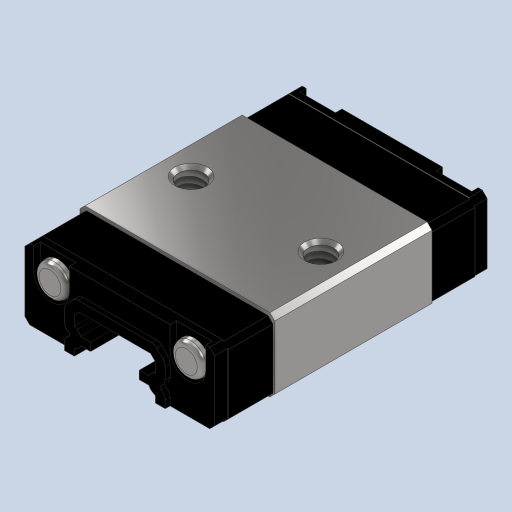
# Autodesk Inventor part: SSEB6_b
Saved by Autodesk Inventor 2023 (Build 270158000, 158)
## iProperties
Category: PARTsolutions
Company: MISUMI
Created: 2024-12-17
Part Number: SSEB6_b
Material: ステンレス鋼
Catalog Web Link: www.cadenas.de
Description: SSEB, SSEB-MX, SSEBV, SSEBV-MX, SSE2B, SSE2B-MX, SSE2BV, SSE2BV-MX, SSEBL, SSEBL-MX, SSEBLV, SSEBLV-MX, SSE2BL, SSE2BL-MX, SSE2BLV, SSE2BLV-MX, SEB, SEBV, SE2B, SE2BV, SEBL, SEBLV, SE2BL, SE2BLV_block-Miniature Linear Guides - Short Block, Standard Preload - High/Precision Grade
Vendor: MISUMI
Document SubType Name: Modeling
Designer: psAdmin
Manufacturer: MISUMI
Mass: 5.50515 g
Surface Area: 8.12596 cm^2
Volume: 0.688144 cm^3
Density: 8 g/cm^3
Appearance: 半つや出し
PSOL_IDENT_0: {$CADENAS_DATA/23d-libs/misumi/metric/06_linear_guides/seb_series/seb_block.prj},358 {VTYP=3D},{NB=S
PSOL_IDENT_1: SEB6_b},{LINA=SSEB6},{NN=SSEB, SSEB-MX, SSEBV, SSEBV-MX, SSE2B, SSE2B-MX, SSE2BV, SSE2BV-MX, SSEBL,
PSOL_IDENT_2: SSEBL-MX, SSEBLV, SSEBLV-MX, SSE2BL, SSE2BL-MX, SSE2BLV, SSE2BLV-MX, SEB, SEBV, SE2B, SE2BV, SEBL, S
PSOL_IDENT_3: EBLV, SE2BL, SE2BLV_block},{DATE=01.06.2021 05:33:03},{GEOMDATE=29.09.2020 01:45:00},{VERSION=},{LIN
PSOL_IDENT_4: EID=60},{WBVAR=TS,MAT,ST,MX},{WBNUMERIC=}  {NB=SSEB6_b},{LINA=SSEB6},{KT=DUMMY},{PN=SSEB6},{TS=},{TY
PSOL_IDENT_5: PE=SSEB},{H=6},{MAT=S},{ST=S},{ST1='S', 'w/o Surface Treatment'},{HARD=56HRC~},{STPN=S},{MX=},{MXALG=
PSOL_IDENT_6: '','w/o MX(Lubrication unit)' },{W=12},{L1=17.4},{B=8},{C=0},{SLL=M2x1.5},{S=2},{LL=1.5},{L2=9.7},{
PSOL_IDENT_7: K=4.5},{CBB=0.3},{W1=5},{W2=3.5},{H1=4.0},{CAA=0.3},{F=15},{G=5.0},{CA1=0.3},{CA2=0.3},{VA1=1.5},{HA
PSOL_IDENT_8: 1=1.0},{WA1=1.2167},{WA2=0.5},{RA1=1.00},{HA2=5.1372},{POIA1=-0.1473},{BHA1=8.4},{BHA2=11.7},{BHA3=1
PSOL_IDENT_9: 1.8},{BHA5=0.0000},{BHA6=0.0},{BHA7=0.0},{BHA8=0.0},{BVA1=1.52},{BVA3=0.15},{BVA4=0.15},{BVA5=4.35},
PSOL_IDENT_10: {BVA6=4.35},{BCA1=0.3},{BCA2H=0.0},{BCA2V=0.00},{BRA1=1.10},{BRA2=1.00},{BDA1=0.00},{BHB1=6.2064},{B
PSOL_IDENT_11: HB2=5.1826},{BVB1=3.1032},{BVB2=1.0652},{BRB1=0.0},{BRB2=0.4732},{BRB3=0.3},{BHC1=2.75},{BHC2=0.8},{
PSOL_IDENT_12: BHC3=0.5},{BHC4=0.4},{BHC5=0.3},{MD=2.3}
NB: SSEB6_b
NN: SSEB, SSEB-MX, SSEBV, SSEBV-MX, SSE2B, SSE2B-MX, SSE2BV, SSE2BV-MX, SSEBL, SSEBL-MX, SSEBLV, SSEBLV-MX, SSE2BL, SSE2BL-MX, SSE2BLV, SSE2BLV-MX, SEB, SEBV, SE2B, SE2BV, SEBL, SEBLV, SE2BL, SE2BLV_block
NT: Miniature Linear Guides - Short Block, Standard Preload - High/Precision Grade
NBSYN: $PN._b
LINA: SSEB6
CATALOG: Misumi
PN: SSEB6
TS: Advanced
H: 6
MAT: Stainless Steel
ST: w/o Surface Treatment
MX: w/o MX(Lubrication unit)
W: 12
L1: 17.4
B: 8
C: 0
SLL: M2x1.5
S: 2
LL: 1.5
L2: 9.7
K: 4.5
CBB: 0.3
W1: 5
W2: 3.5
H1: 4
CAA: 0.3
F: 15
G: 5
CA1: 0.3
CA2: 0.3
VA1: 1.5
HA1: 1
WA1: 1.2167
WA2: 0.5
RA1: 1
HA2: 5.1372
POIA1: -0.1473
BHA1: 8.4
BHA2: 11.7
BHA3: 11.8
BHA5: 0
BHA6: 0
BHA7: 0
BHA8: 0
BVA1: 1.52
BVA3: 0.15
BVA4: 0.15
BVA5: 4.35
BVA6: 4.35
BCA1: 0.3
BCA2H: 0
BCA2V: 0
BRA1: 1.1
BRA2: 1
BDA1: 0
BHB1: 6.2064
BHB2: 5.1826
BVB1: 3.1032
BVB2: 1.0652
BRB1: 0
BRB2: 0.4732
BRB3: 0.3
BHC1: 2.75
BHC2: 0.8
BHC3: 0.5
BHC4: 0.4
BHC5: 0.3
MD: 2.3
SUPPLIER: MISUMI
ARTICLENO: SSEB6_b
BOMINFO: SSEB6
CREATOR: CADENAS GmbH
Title: SSEB6
Author: Cadenas PARTsolutions
Comments: Miniature Linear Guides - Short Block, Standard Preload - High/Precision Grade
Autodesk Inventor part; units mm, degrees
sketch "Sketch_29" plane through (0, 0, 0) normal (0, 0, 1) x (1, 0, 0)
  line L0 (-6, 1.8) -> (-5.7, 1.5)
  line L1 (-5.7, 1.5) -> (5.7, 1.5)
  line L2 (5.7, 1.5) -> (6, 1.8)
  line L3 (6, 1.8) -> (6, 5.7)
  line L4 (6, 5.7) -> (5.7, 6)
  line L5 (5.7, 6) -> (-5.7, 6)
  line L6 (-5.7, 6) -> (-6, 5.7)
  line L7 (-6, 5.7) -> (-6, 1.8)
  constraints: 16 end point
extrude "Extrusion1" add sketch "Sketch_29" along normal mid plane 9.7
sketch "Sketch_3" plane through (0, 0, 4.85) normal (0, 0, 1) x (1, 0, 0)
  line L0 (-5.9, 5.55) -> (-5.9, 1.8)
  line L1 (-5.9, 1.8) -> (-5.6, 1.5)
  line L2 (-5.6, 1.5) -> (5.6, 1.5)
  line L3 (5.6, 1.5) -> (5.9, 1.8)
  line L4 (5.9, 1.8) -> (5.9, 5.55)
  line L5 (5.9, 5.55) -> (5.6, 5.85)
  line L6 (5.6, 5.85) -> (-5.6, 5.85)
  line L7 (-5.6, 5.85) -> (-5.9, 5.55)
  constraints: 16 end point
extrude "Extrusion2" add sketch "Sketch_3" along normal blind 3.85
sketch "Sketch_42" plane through (0, 0, 4.85) normal (0, 0, 1) x (1, 0, 0)
  line L0 (-12, 7.2) -> (-12, 0)
  line L1 (-12, 0) -> (12, 0)
  line L2 (12, 0) -> (12, 7.2)
  line L3 (12, 7.2) -> (-12, 7.2)
  line L4 (-5.9, 5.5) -> (-5.9, 1.8)
  line L5 (-5.9, 1.8) -> (-5.6, 1.5)
  line L6 (-5.6, 1.5) -> (5.6, 1.5)
  line L7 (5.6, 1.5) -> (5.9, 1.8)
  line L8 (5.9, 1.8) -> (5.9, 5.5)
  line L9 (5.9, 5.5) -> (5.6, 5.8)
  line L10 (5.6, 5.8) -> (-5.6, 5.8)
  line L11 (-5.6, 5.8) -> (-5.9, 5.5)
  constraints: 24 end point
extrude "Extrusion3" cut sketch "Sketch_42" along normal blind 2.75
sketch "Sketch_4" plane through (0, 0, -4.85) normal (0, 0, 1) x (1, 0, 0)
  line L0 (-5.9, 5.55) -> (-5.9, 1.8)
  line L1 (-5.9, 1.8) -> (-5.6, 1.5)
  line L2 (-5.6, 1.5) -> (5.6, 1.5)
  line L3 (5.6, 1.5) -> (5.9, 1.8)
  line L4 (5.9, 1.8) -> (5.9, 5.55)
  line L5 (5.9, 5.55) -> (5.6, 5.85)
  line L6 (5.6, 5.85) -> (-5.6, 5.85)
  line L7 (-5.6, 5.85) -> (-5.9, 5.55)
  constraints: 16 end point
extrude "Extrusion4" add sketch "Sketch_4" against normal blind 3.85
sketch "Sketch_43" plane through (0, 0, -4.85) normal (0, 0, 1) x (1, 0, 0)
  line L0 (-12, 7.2) -> (-12, 0)
  line L1 (-12, 0) -> (12, 0)
  line L2 (12, 0) -> (12, 7.2)
  line L3 (12, 7.2) -> (-12, 7.2)
  line L4 (-5.9, 5.5) -> (-5.9, 1.8)
  line L5 (-5.9, 1.8) -> (-5.6, 1.5)
  line L6 (-5.6, 1.5) -> (5.6, 1.5)
  line L7 (5.6, 1.5) -> (5.9, 1.8)
  line L8 (5.9, 1.8) -> (5.9, 5.5)
  line L9 (5.9, 5.5) -> (5.6, 5.8)
  line L10 (5.6, 5.8) -> (-5.6, 5.8)
  line L11 (-5.6, 5.8) -> (-5.9, 5.5)
  constraints: 24 end point
extrude "Extrusion5" cut sketch "Sketch_43" against normal blind 2.75
sketch "Sketch_30" plane through (0, 0, 8.7) normal (0, 0, 1) x (1, 0, 0)
  line L0 (-12, 9) -> (-12, 0)
  line L1 (-12, 0) -> (12, 0)
  line L2 (12, 0) -> (12, 9)
  line L3 (12, 9) -> (-12, 9)
  line L4 (-5.85, 1.8) -> (-5.55, 1.5)
  line L5 (-5.55, 1.5) -> (5.55, 1.5)
  line L6 (5.55, 1.5) -> (5.85, 1.8)
  line L7 (5.85, 1.8) -> (5.85, 5.55)
  line L8 (5.85, 5.55) -> (5.55, 5.85)
  line L9 (5.55, 5.85) -> (5.3, 5.85)
  line L10 (5.3, 5.85) -> (5.3, 4.48)
  arc A0 (3.1, 4.48) -> (5.3, 4.48) centre (4.2, 4.48) ccw
  line L11 (3.1, 4.48) -> (3.1, 5.85)
  line L12 (3.1, 5.85) -> (-3.1, 5.85)
  line L13 (-3.1, 5.85) -> (-3.1, 4.48)
  arc A1 (-5.3, 4.48) -> (-3.1, 4.48) centre (-4.2, 4.48) ccw
  line L14 (-5.3, 4.48) -> (-5.3, 5.85)
  line L15 (-5.3, 5.85) -> (-5.55, 5.85)
  line L16 (-5.55, 5.85) -> (-5.85, 5.55)
  line L17 (-5.85, 5.55) -> (-5.85, 1.8)
  constraints: 36 end point, 4 point on circle, 2 centre point
extrude "Extrusion6" cut sketch "Sketch_30" against normal blind 1.1
sketch "_____2" plane through (0, 0, 8.7) normal (0, 0, 1) x (1, 0, 0)
  line L0 (-12, 7.2) -> (-12, 0)
  line L1 (-12, 0) -> (-3.1032, 0)
  line L2 (-3.1032, 0) -> (-3.1032, 1.9674)
  arc A0 (-2.8479, 2.3874) -> (-3.1032, 1.9674) centre (-2.63, 1.9674) ccw
  arc A1 (-2.8479, 2.3874) -> (-2.8479, 2.6126) centre (-2.9063, 2.5) ccw
  arc A2 (-3.1032, 3.0326) -> (-2.8479, 2.6126) centre (-2.63, 3.0326) ccw
  line L3 (-3.1032, 3.0326) -> (-3.1032, 3.7539)
  arc A3 (-2.9646, 4.0885) -> (-3.1032, 3.7539) centre (-2.63, 3.7539) ccw
  line L4 (-2.9646, 4.0885) -> (-2.5885, 4.4646)
  arc A4 (-2.2539, 4.6032) -> (-2.5885, 4.4646) centre (-2.2539, 4.13) ccw
  line L5 (-2.2539, 4.6032) -> (2.2539, 4.6032)
  arc A5 (2.5885, 4.4646) -> (2.2539, 4.6032) centre (2.2539, 4.13) ccw
  line L6 (2.5885, 4.4646) -> (2.9646, 4.0885)
  arc A6 (3.1032, 3.7539) -> (2.9646, 4.0885) centre (2.63, 3.7539) ccw
  line L7 (3.1032, 3.7539) -> (3.1032, 3.0326)
  arc A7 (2.8479, 2.6126) -> (3.1032, 3.0326) centre (2.63, 3.0326) ccw
  arc A8 (2.8479, 2.6126) -> (2.8479, 2.3874) centre (2.9063, 2.5) ccw
  arc A9 (3.1032, 1.9674) -> (2.8479, 2.3874) centre (2.63, 1.9674) ccw
  line L8 (3.1032, 1.9674) -> (3.1032, 0)
  line L9 (3.1032, 0) -> (12, 0)
  line L10 (12, 0) -> (12, 7.2)
  line L11 (12, 7.2) -> (-12, 7.2)
  constraints: 24 end point, 20 point on circle, 10 centre point
extrude "Extrusion7" cut sketch "_____2" against normal blind 0.3
sketch "Sketch_31" plane through (0, 0, -8.7) normal (0, 0, 1) x (1, 0, 0)
  line L0 (-12, 9) -> (-12, 0)
  line L1 (-12, 0) -> (12, 0)
  line L2 (12, 0) -> (12, 9)
  line L3 (12, 9) -> (-12, 9)
  line L4 (-5.85, 1.8) -> (-5.55, 1.5)
  line L5 (-5.55, 1.5) -> (5.55, 1.5)
  line L6 (5.55, 1.5) -> (5.85, 1.8)
  line L7 (5.85, 1.8) -> (5.85, 5.55)
  line L8 (5.85, 5.55) -> (5.55, 5.85)
  line L9 (5.55, 5.85) -> (5.3, 5.85)
  line L10 (5.3, 5.85) -> (5.3, 4.48)
  arc A0 (3.1, 4.48) -> (5.3, 4.48) centre (4.2, 4.48) ccw
  line L11 (3.1, 4.48) -> (3.1, 5.85)
  line L12 (3.1, 5.85) -> (-3.1, 5.85)
  line L13 (-3.1, 5.85) -> (-3.1, 4.48)
  arc A1 (-5.3, 4.48) -> (-3.1, 4.48) centre (-4.2, 4.48) ccw
  line L14 (-5.3, 4.48) -> (-5.3, 5.85)
  line L15 (-5.3, 5.85) -> (-5.55, 5.85)
  line L16 (-5.55, 5.85) -> (-5.85, 5.55)
  line L17 (-5.85, 5.55) -> (-5.85, 1.8)
  constraints: 36 end point, 4 point on circle, 2 centre point
extrude "Extrusion8" cut sketch "Sketch_31" along normal blind 1.1
sketch "_____1" plane through (0, 0, -8.7) normal (0, 0, 1) x (1, 0, 0)
  line L0 (-12, 7.2) -> (-12, 0)
  line L1 (-12, 0) -> (-3.1032, 0)
  line L2 (-3.1032, 0) -> (-3.1032, 1.9674)
  arc A0 (-2.8479, 2.3874) -> (-3.1032, 1.9674) centre (-2.63, 1.9674) ccw
  arc A1 (-2.8479, 2.3874) -> (-2.8479, 2.6126) centre (-2.9063, 2.5) ccw
  arc A2 (-3.1032, 3.0326) -> (-2.8479, 2.6126) centre (-2.63, 3.0326) ccw
  line L3 (-3.1032, 3.0326) -> (-3.1032, 3.7539)
  arc A3 (-2.9646, 4.0885) -> (-3.1032, 3.7539) centre (-2.63, 3.7539) ccw
  line L4 (-2.9646, 4.0885) -> (-2.5885, 4.4646)
  arc A4 (-2.2539, 4.6032) -> (-2.5885, 4.4646) centre (-2.2539, 4.13) ccw
  line L5 (-2.2539, 4.6032) -> (2.2539, 4.6032)
  arc A5 (2.5885, 4.4646) -> (2.2539, 4.6032) centre (2.2539, 4.13) ccw
  line L6 (2.5885, 4.4646) -> (2.9646, 4.0885)
  arc A6 (3.1032, 3.7539) -> (2.9646, 4.0885) centre (2.63, 3.7539) ccw
  line L7 (3.1032, 3.7539) -> (3.1032, 3.0326)
  arc A7 (2.8479, 2.6126) -> (3.1032, 3.0326) centre (2.63, 3.0326) ccw
  arc A8 (2.8479, 2.6126) -> (2.8479, 2.3874) centre (2.9063, 2.5) ccw
  arc A9 (3.1032, 1.9674) -> (2.8479, 2.3874) centre (2.63, 1.9674) ccw
  line L8 (3.1032, 1.9674) -> (3.1032, 0)
  line L9 (3.1032, 0) -> (12, 0)
  line L10 (12, 0) -> (12, 7.2)
  line L11 (12, 7.2) -> (-12, 7.2)
  constraints: 24 end point, 20 point on circle, 10 centre point
extrude "Extrusion9" cut sketch "_____1" along normal blind 0.3
sketch "Sketch_32" plane through (0, 0, 7.6) normal (0, 0, 1) x (1, 0, 0)
  arc A0 (-5.3, 4.48) -> (-3.1, 4.48) centre (-4.2, 4.48) ccw
  line L0 (-3.1, 4.48) -> (-3.1, 5.85)
  line L1 (-3.1, 5.85) -> (-5.3, 5.85)
  line L2 (-5.3, 5.85) -> (-5.3, 4.48)
  constraints: 6 end point, 2 point on circle, 1 centre point
extrude "Extrusion10" add sketch "Sketch_32" along normal blind 0.4
sketch "Sketch_33" plane through (0, 0, 7.6) normal (0, 0, 1) x (1, 0, 0)
  arc A0 (3.1, 4.48) -> (5.3, 4.48) centre (4.2, 4.48) ccw
  line L0 (5.3, 4.48) -> (5.3, 5.85)
  line L1 (5.3, 5.85) -> (3.1, 5.85)
  line L2 (3.1, 5.85) -> (3.1, 4.48)
  constraints: 6 end point, 2 point on circle, 1 centre point
extrude "Extrusion11" add sketch "Sketch_33" along normal blind 0.4
sketch "Sketch_34" plane through (0, 0, -7.6) normal (0, 0, 1) x (1, 0, 0)
  arc A0 (-5.3, 4.48) -> (-3.1, 4.48) centre (-4.2, 4.48) ccw
  line L0 (-3.1, 4.48) -> (-3.1, 5.85)
  line L1 (-3.1, 5.85) -> (-5.3, 5.85)
  line L2 (-5.3, 5.85) -> (-5.3, 4.48)
  constraints: 6 end point, 2 point on circle, 1 centre point
extrude "Extrusion12" add sketch "Sketch_34" against normal blind 0.4
sketch "Sketch_35" plane through (0, 0, -7.6) normal (0, 0, 1) x (1, 0, 0)
  arc A0 (3.1, 4.48) -> (5.3, 4.48) centre (4.2, 4.48) ccw
  line L0 (5.3, 4.48) -> (5.3, 5.85)
  line L1 (5.3, 5.85) -> (3.1, 5.85)
  line L2 (3.1, 5.85) -> (3.1, 4.48)
  constraints: 6 end point, 2 point on circle, 1 centre point
extrude "Extrusion13" add sketch "Sketch_35" against normal blind 0.4
sketch "Sketch_36" plane through (-4.2, 0, 0) normal (1, 0, 0) x (0, 0, -1)
  line L0 (-8, 4.48) -> (-8.5, 4.48)
  line L1 (-8.5, 4.48) -> (-8.5, 5.1602)
  arc A0 (-8.2277, 5.4589) -> (-8.5, 5.1602) centre (-8.2, 5.1602) ccw
  line L2 (-8.2277, 5.4589) -> (-8, 5.48)
  line L3 (-8, 5.48) -> (-8, 4.48)
  line L4 (-8, 4.48) -> (-8.5, 4.48)
  constraints: 10 end point, 2 point on circle, 1 centre point
revolve "Revolution1" add sketch "Sketch_36" angle 360 about axis through (-4.2, 4.48, 8) along (0, 0, -1)
sketch "Sketch_37" plane through (-4.2, 0, 0) normal (1, 0, 0) x (0, 0, -1)
  line L0 (8.5, 4.48) -> (8, 4.48)
  line L1 (8, 4.48) -> (8, 5.48)
  line L2 (8, 5.48) -> (8.2277, 5.4589)
  arc A0 (8.5, 5.1602) -> (8.2277, 5.4589) centre (8.2, 5.1602) ccw
  line L3 (8.5, 5.1602) -> (8.5, 4.48)
  line L4 (8.5, 4.48) -> (8, 4.48)
  constraints: 10 end point, 2 point on circle, 1 centre point
revolve "Revolution2" add sketch "Sketch_37" angle 360 about axis through (-4.2, 4.48, -8.5) along (0, 0, -1)
sketch "Sketch_38" plane through (4.2, 0, 0) normal (1, 0, 0) x (0, 0, -1)
  line L0 (-8, 4.48) -> (-8.5, 4.48)
  line L1 (-8.5, 4.48) -> (-8.5, 5.1602)
  arc A0 (-8.2277, 5.4589) -> (-8.5, 5.1602) centre (-8.2, 5.1602) ccw
  line L2 (-8.2277, 5.4589) -> (-8, 5.48)
  line L3 (-8, 5.48) -> (-8, 4.48)
  line L4 (-8, 4.48) -> (-8.5, 4.48)
  constraints: 10 end point, 2 point on circle, 1 centre point
revolve "Revolution3" add sketch "Sketch_38" angle 360 about axis through (4.2, 4.48, 8) along (0, 0, -1)
sketch "Sketch_39" plane through (4.2, 0, 0) normal (1, 0, 0) x (0, 0, -1)
  line L0 (8.5, 4.48) -> (8, 4.48)
  line L1 (8, 4.48) -> (8, 5.48)
  line L2 (8, 5.48) -> (8.2277, 5.4589)
  arc A0 (8.5, 5.1602) -> (8.2277, 5.4589) centre (8.2, 5.1602) ccw
  line L3 (8.5, 5.1602) -> (8.5, 4.48)
  line L4 (8.5, 4.48) -> (8, 4.48)
  constraints: 10 end point, 2 point on circle, 1 centre point
revolve "Revolution4" add sketch "Sketch_39" angle 360 about axis through (4.2, 4.48, -8.5) along (0, 0, -1)
sketch "Sketch_17" plane through (0, 0, 0) normal (0, 0, 1) x (1, 0, 0)
  line L0 (-2.5, 3.7) -> (-2.5, 3.1084)
  line L1 (-2.5, 3.1084) -> (-2.3242, 3.0098)
  arc A0 (-2.1007, 2.75) -> (-2.3242, 3.0098) centre (-2.5686, 2.5736) ccw
  line L2 (-2.1007, 2.75) -> (-1.5, 2.75)
  line L3 (-1.5, 2.75) -> (-1.5, 2.25)
  line L4 (-1.5, 2.25) -> (-2.1007, 2.25)
  arc A1 (-2.3242, 1.9902) -> (-2.1007, 2.25) centre (-2.5686, 2.4264) ccw
  line L5 (-2.3242, 1.9902) -> (-2.5, 1.8917)
  line L6 (-2.5, 1.8917) -> (-2.5, 0.3)
  line L7 (-2.5, 0.3) -> (-2.2, 0)
  line L8 (-2.2, 0) -> (2.2, 0)
  line L9 (2.2, 0) -> (2.5, 0.3)
  line L10 (2.5, 0.3) -> (2.5, 1.8917)
  line L11 (2.5, 1.8917) -> (2.3242, 1.9902)
  arc A2 (2.1007, 2.25) -> (2.3242, 1.9902) centre (2.5686, 2.4263) ccw
  line L12 (2.1007, 2.25) -> (1.5, 2.25)
  line L13 (1.5, 2.25) -> (1.5, 2.75)
  line L14 (1.5, 2.75) -> (2.1007, 2.75)
  arc A3 (2.3242, 3.0098) -> (2.1007, 2.75) centre (2.5686, 2.5737) ccw
  line L15 (2.3242, 3.0098) -> (2.5, 3.1084)
  line L16 (2.5, 3.1084) -> (2.5, 3.7)
  line L17 (2.5, 3.7) -> (2.2, 4)
  line L18 (2.2, 4) -> (-2.2, 4)
  line L19 (-2.2, 4) -> (-2.5, 3.7)
  constraints: 40 end point, 8 point on circle, 4 centre point
extrude "Extrusion14" cut sketch "Sketch_17" along normal mid plane 9.7
sketch "Sketch_11" plane through (0, 0, 4.85) normal (0, 0, 1) x (1, 0, 0)
  line L0 (-2.5, 3.7) -> (-2.5, 3.1084)
  line L1 (-2.5, 3.1084) -> (-2.3242, 3.0098)
  arc A0 (-2.1007, 2.75) -> (-2.3242, 3.0098) centre (-2.5686, 2.5736) ccw
  line L2 (-2.1007, 2.75) -> (-1.5, 2.75)
  line L3 (-1.5, 2.75) -> (-1.5, 2.25)
  line L4 (-1.5, 2.25) -> (-2.1007, 2.25)
  arc A1 (-2.3242, 1.9902) -> (-2.1007, 2.25) centre (-2.5686, 2.4264) ccw
  line L5 (-2.3242, 1.9902) -> (-2.5, 1.8917)
  line L6 (-2.5, 1.8917) -> (-2.5, 0.3)
  line L7 (-2.5, 0.3) -> (-2.2, 0)
  line L8 (-2.2, 0) -> (2.2, 0)
  line L9 (2.2, 0) -> (2.5, 0.3)
  line L10 (2.5, 0.3) -> (2.5, 1.8917)
  line L11 (2.5, 1.8917) -> (2.3242, 1.9902)
  arc A2 (2.1007, 2.25) -> (2.3242, 1.9902) centre (2.5686, 2.4263) ccw
  line L12 (2.1007, 2.25) -> (1.5, 2.25)
  line L13 (1.5, 2.25) -> (1.5, 2.75)
  line L14 (1.5, 2.75) -> (2.1007, 2.75)
  arc A3 (2.3242, 3.0098) -> (2.1007, 2.75) centre (2.5686, 2.5737) ccw
  line L15 (2.3242, 3.0098) -> (2.5, 3.1084)
  line L16 (2.5, 3.1084) -> (2.5, 3.7)
  line L17 (2.5, 3.7) -> (2.2, 4)
  line L18 (2.2, 4) -> (-2.2, 4)
  line L19 (-2.2, 4) -> (-2.5, 3.7)
  constraints: 40 end point, 8 point on circle, 4 centre point
extrude "Extrusion15" cut sketch "Sketch_11" along normal blind 4.85
sketch "Sketch_22" plane through (0, 0, 4.85) normal (0, 0, 1) x (1, 0, 0)
  line L0 (-12, 9) -> (-12, 0)
  line L1 (-12, 0) -> (12, 0)
  line L2 (12, 0) -> (12, 9)
  line L3 (12, 9) -> (-12, 9)
  line L4 (-5.9, 5.6) -> (-5.9, 1.8)
  line L5 (-5.9, 1.8) -> (-5.65, 1.55)
  line L6 (-5.65, 1.55) -> (-2.55, 1.55)
  line L7 (-2.55, 1.55) -> (-2.55, 1.9417)
  line L8 (-2.55, 1.9417) -> (-2.3847, 2.0156)
  arc A0 (-2.3847, 2.0156) -> (-2.1367, 2.3) centre (-2.5686, 2.4263) ccw
  line L9 (-2.1367, 2.3) -> (-1.55, 2.3)
  line L10 (-1.55, 2.3) -> (-1.55, 2.7)
  line L11 (-1.55, 2.7) -> (-2.1367, 2.7)
  arc A1 (-2.1367, 2.7) -> (-2.3847, 2.9844) centre (-2.5686, 2.5737) ccw
  line L12 (-2.3847, 2.9844) -> (-2.55, 3.0584)
  line L13 (-2.55, 3.0584) -> (-2.55, 3.75)
  line L14 (-2.55, 3.75) -> (-2.25, 4.05)
  line L15 (-2.25, 4.05) -> (2.25, 4.05)
  line L16 (2.25, 4.05) -> (2.55, 3.75)
  line L17 (2.55, 3.75) -> (2.55, 3.0584)
  line L18 (2.55, 3.0584) -> (2.3847, 2.9844)
  arc A2 (2.3847, 2.9844) -> (2.1367, 2.7) centre (2.5686, 2.5737) ccw
  line L19 (2.1367, 2.7) -> (1.55, 2.7)
  line L20 (1.55, 2.7) -> (1.55, 2.3)
  line L21 (1.55, 2.3) -> (2.1367, 2.3)
  arc A3 (2.1367, 2.3) -> (2.3847, 2.0156) centre (2.5686, 2.4263) ccw
  line L22 (2.3847, 2.0156) -> (2.55, 1.9417)
  line L23 (2.55, 1.9417) -> (2.55, 1.55)
  line L24 (2.55, 1.55) -> (5.65, 1.55)
  line L25 (5.65, 1.55) -> (5.9, 1.8)
  line L26 (5.9, 1.8) -> (5.9, 5.6)
  line L27 (5.9, 5.6) -> (5.65, 5.85)
  line L28 (5.65, 5.85) -> (-5.65, 5.85)
  line L29 (-5.65, 5.85) -> (-5.9, 5.6)
  constraints: 60 end point, 8 point on circle, 4 centre point
extrude "Extrusion16" cut sketch "Sketch_22" along normal blind 0.05
sketch "Sketch_10" plane through (0, 0, -4.85) normal (0, 0, 1) x (1, 0, 0)
  line L0 (-2.5, 3.7) -> (-2.5, 3.1084)
  line L1 (-2.5, 3.1084) -> (-2.3242, 3.0098)
  arc A0 (-2.1007, 2.75) -> (-2.3242, 3.0098) centre (-2.5686, 2.5736) ccw
  line L2 (-2.1007, 2.75) -> (-1.5, 2.75)
  line L3 (-1.5, 2.75) -> (-1.5, 2.25)
  line L4 (-1.5, 2.25) -> (-2.1007, 2.25)
  arc A1 (-2.3242, 1.9902) -> (-2.1007, 2.25) centre (-2.5686, 2.4264) ccw
  line L5 (-2.3242, 1.9902) -> (-2.5, 1.8917)
  line L6 (-2.5, 1.8917) -> (-2.5, 0.3)
  line L7 (-2.5, 0.3) -> (-2.2, 0)
  line L8 (-2.2, 0) -> (2.2, 0)
  line L9 (2.2, 0) -> (2.5, 0.3)
  line L10 (2.5, 0.3) -> (2.5, 1.8917)
  line L11 (2.5, 1.8917) -> (2.3242, 1.9902)
  arc A2 (2.1007, 2.25) -> (2.3242, 1.9902) centre (2.5686, 2.4263) ccw
  line L12 (2.1007, 2.25) -> (1.5, 2.25)
  line L13 (1.5, 2.25) -> (1.5, 2.75)
  line L14 (1.5, 2.75) -> (2.1007, 2.75)
  arc A3 (2.3242, 3.0098) -> (2.1007, 2.75) centre (2.5686, 2.5737) ccw
  line L15 (2.3242, 3.0098) -> (2.5, 3.1084)
  line L16 (2.5, 3.1084) -> (2.5, 3.7)
  line L17 (2.5, 3.7) -> (2.2, 4)
  line L18 (2.2, 4) -> (-2.2, 4)
  line L19 (-2.2, 4) -> (-2.5, 3.7)
  constraints: 40 end point, 8 point on circle, 4 centre point
extrude "Extrusion17" cut sketch "Sketch_10" against normal blind 4.85
sketch "Sketch_23" plane through (0, 0, -4.85) normal (0, 0, 1) x (1, 0, 0)
  line L0 (-12, 9) -> (-12, 0)
  line L1 (-12, 0) -> (12, 0)
  line L2 (12, 0) -> (12, 9)
  line L3 (12, 9) -> (-12, 9)
  line L4 (-5.9, 5.6) -> (-5.9, 1.8)
  line L5 (-5.9, 1.8) -> (-5.65, 1.55)
  line L6 (-5.65, 1.55) -> (-2.55, 1.55)
  line L7 (-2.55, 1.55) -> (-2.55, 1.9417)
  line L8 (-2.55, 1.9417) -> (-2.3847, 2.0156)
  arc A0 (-2.3847, 2.0156) -> (-2.1367, 2.3) centre (-2.5686, 2.4263) ccw
  line L9 (-2.1367, 2.3) -> (-1.55, 2.3)
  line L10 (-1.55, 2.3) -> (-1.55, 2.7)
  line L11 (-1.55, 2.7) -> (-2.1367, 2.7)
  arc A1 (-2.1367, 2.7) -> (-2.3847, 2.9844) centre (-2.5686, 2.5737) ccw
  line L12 (-2.3847, 2.9844) -> (-2.55, 3.0584)
  line L13 (-2.55, 3.0584) -> (-2.55, 3.75)
  line L14 (-2.55, 3.75) -> (-2.25, 4.05)
  line L15 (-2.25, 4.05) -> (2.25, 4.05)
  line L16 (2.25, 4.05) -> (2.55, 3.75)
  line L17 (2.55, 3.75) -> (2.55, 3.0584)
  line L18 (2.55, 3.0584) -> (2.3847, 2.9844)
  arc A2 (2.3847, 2.9844) -> (2.1367, 2.7) centre (2.5686, 2.5737) ccw
  line L19 (2.1367, 2.7) -> (1.55, 2.7)
  line L20 (1.55, 2.7) -> (1.55, 2.3)
  line L21 (1.55, 2.3) -> (2.1367, 2.3)
  arc A3 (2.1367, 2.3) -> (2.3847, 2.0156) centre (2.5686, 2.4263) ccw
  line L22 (2.3847, 2.0156) -> (2.55, 1.9417)
  line L23 (2.55, 1.9417) -> (2.55, 1.55)
  line L24 (2.55, 1.55) -> (5.65, 1.55)
  line L25 (5.65, 1.55) -> (5.9, 1.8)
  line L26 (5.9, 1.8) -> (5.9, 5.6)
  line L27 (5.9, 5.6) -> (5.65, 5.85)
  line L28 (5.65, 5.85) -> (-5.65, 5.85)
  line L29 (-5.65, 5.85) -> (-5.9, 5.6)
  constraints: 60 end point, 8 point on circle, 4 centre point
extrude "Extrusion18" cut sketch "Sketch_23" against normal blind 0.05
sketch "Sketch23" plane through (-5.7, 6, 4.85) normal (0, 1, 0) x (1, 0, 0)
  point P0 (1.7, 4.85)
hole "Hole1" at (-4, 6, 0) direction (0, -1, 0) diameter 1.567 depth 2.3 tip angle 120 countersink diameter 2 countersink angle 90 thread size "M2x0.4" class "6H" standard "ISO Metric profile"
pattern_linear "Rectangular Pattern1" count 2 spacing 8 along (1, 0, 0) of "Hole1"
ref_plane "to_rail_XY" through (0, 4, 0) normal (0, 0, 1) x (1, 0, 0)
ref_plane "to_rail_YZ" through (0, 4, 0) normal (1, 0, 0) x (0, 1, 0)
ref_plane "to_rail_ZX" through (0, 4, 0) normal (0, 1, 0) x (0, 0, 1)
body "Solid1"
